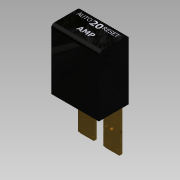
# Autodesk Inventor part: VB3-A20-F57
Saved by Autodesk Inventor 2020.1 (Build 241239000, 239)
## iProperties
Created: 2019-11-19
Part Number: VB3-A20-F57
Document SubType Name: Modeling
Designer: Autodesk Inc.
Density: 1 g/cm^3
Catalog Web Link: http://www.snapaction.net/pdf/vb3.pdf
Description: Circuit Breaker 20 Amp
Vendor: Snap Action
Material: Generic
Appearance: Glossy - Black
Category: Bag #3
Company: Autodesk Inc.
Author: Autodesk Inc.
Keywords: Black Tote
Autodesk Inventor part; units mm, degrees
note: some values were not read from the file. Chosen so that the rebuilt part matches the saved one: direction of "Emboss1"; direction of "Emboss3".
sketch "Sketch1" plane through (0, 0, 0) normal (0, 0, 1) x (1, 0, 0)
  line L0 (0, 0) -> (15.748, 0)
  line L1 (15.748, 0) -> (15.748, 9.906)
  line L2 (15.748, 9.906) -> (0, 9.906)
  line L3 (0, 9.906) -> (0, 0)
  dimension "d0" = 15.748
  dimension "d1" = 9.906
  constraints: 8 end point, 2 parallel, 1 horizontal, 1 perpendicular
  measures "d0" distance of L1.end L2.end
  measures "d1" distance of L0.end L1.end
extrude "Extrusion1" add sketch "Sketch1" against normal blind 19.812
fillet "Fillet1" radius 0.254 8 edges at (0, 0, -9.906) (15.748, 0, -9.906) (15.748, 9.906, -9.906) (0, 9.906, -9.906) (7.874, 0, -19.812) (7.874, 9.906, -19.812) (15.748, 4.953, -19.812) (0, 4.953, -19.812)
fillet "Fillet1" radius 1.27 2 edges at (7.874, 0, 0) (7.874, 9.906, 0)
sketch "Sketch2" plane through (0, 0, -19.812) normal (0, 0, -1) x (-1, 0, 0)
  line L0 (-1.0033, 8.6678) -> (-6.3881, 8.6677)
  line L1 (-6.3881, 8.6677) -> (-6.3881, 7.8803)
  line L2 (-6.3881, 7.8803) -> (-1.0033, 7.8803)
  line L3 (-1.0033, 7.8803) -> (-1.0033, 8.6678)
  line L4 (-0.254, 9.906) -> (-15.494, 9.906) projected
  line L5 (-0.254, 0.254) -> (-15.494, 0.254) projected
  line L6 (-15.494, 9.652) -> (-0.254, 9.652) projected
  line L7 (-7.874, 0.254) -> (-7.874, 9.652) construction
  point P0 (0, 0)
  dimension "d6" = 5.3848
  dimension "d8" = 0.7874
  dimension "d13" = 1.4859
  constraints: 10 end point, 2 midpoint, 2 parallel, 1 horizontal, 1 perpendicular
  measures "d6" distance of L1.end L2.end
  measures "d8" distance of L2.end L0.start
  measures "d13" distance between parallel lines of L7 L1
extrude "Extrusion3" add sketch "Sketch2" along normal blind 14.478
sketch "Sketch3" plane through (6.3881, 7.8803, -19.812) normal (1, 0, 0) x (0, 0, -1)
  line L0 (14.478, 0) -> (14.478, 0.7874) projected
  line L1 (0, 0.7874) -> (14.478, 0.7874) projected
  line L2 (0, 0) -> (14.478, 0) projected
  line L3 (13.8941, 0) -> (14.478, 0.3937)
  line L4 (13.8941, 0.7874) -> (14.478, 0.3937)
  point P0 (-19.812, -7.8803)
  constraints: 4 end point, 2 point on line, 1 midpoint
extrude "Extrusion4" cut sketch "Sketch3" against normal up to next
sketch "Sketch4" plane through (1.0033, 7.8803, -19.812) normal (0, -1, 0) x (1, 0, 0)
  line L0 (5.3848, -14.478) -> (0, -14.478) projected
  line L1 (0, -13.8941) -> (0.5839, -14.478)
  line L2 (5.3848, -13.8941) -> (4.8009, -14.478)
  line L3 (0, -13.8941) -> (0, -14.478)
  line L4 (4.8009, -14.478) -> (5.3848, -14.478)
  line L5 (5.3848, -13.8941) -> (5.3848, -14.478)
  point P0 (-1.0033, 19.812)
  dimension "d18" = 0.5839
  dimension "d19" = 0.5839
  dimension "d20" = 0.5839
  constraints: 10 end point, 3 perpendicular, 2 point on line, 1 collinear
  measures "d18" distance of L0.end L1.start
  measures "d19" distance of L1.end L0.end
  measures "d20" distance of L0.start L2.end
extrude "Extrusion5" cut sketch "Sketch4" against normal through all
ref_plane "Work Plane1" through (7.874, 1.27, 0) normal (1, 0, 0) x (0, 0, -1)
mirror "Mirror1" about plane through (7.874, 1.27, 0) normal (1, 0, 0) of "Extrusion3", "Extrusion4", "Extrusion5"
ref_plane "Work Plane2" through (0, 0, 4.7625) normal (0, 0, 1) x (1, 0, 0)
sketch "Sketch6" plane through (0, 0, 4.7625) normal (0, 0, 1) x (1, 0, 0)
  line L0 (-0.5435, 9.1913) -> (16.2915, 9.1913) construction
  line L1 (16.2915, 9.1913) -> (16.2915, 2.8312) construction
  line L2 (16.2915, 2.8312) -> (-0.5435, 2.8312) construction
  line L3 (-0.5435, 2.8312) -> (-0.5435, 9.1913) construction
  line L4 (0, 8.636) -> (15.748, 8.636) projected
  line L5 (1.2137, 7.0222) -> (1.6418, 8.2922)
  line L6 (1.6418, 8.2922) -> (1.8497, 8.2922)
  line L7 (1.8497, 8.2922) -> (2.2779, 7.0222)
  line L8 (2.2779, 7.0222) -> (2.0998, 7.0222)
  line L9 (2.0998, 7.0222) -> (1.9846, 7.3773)
  line L10 (1.9846, 7.3773) -> (1.4998, 7.3773)
  line L11 (1.4998, 7.3773) -> (1.3845, 7.0222)
  line L12 (1.3845, 7.0222) -> (1.2137, 7.0222)
  line L13 (1.9382, 7.5213) -> (1.7417, 8.1193)
  line L14 (1.7417, 8.1193) -> (1.5461, 7.5213)
  line L15 (1.5461, 7.5213) -> (1.9382, 7.5213)
  spline S0 degree 2 poles (2.8419, 6.9954) (2.7297, 6.9954) (2.563, 7.0541) (2.5043, 7.1128) knots 0 0 0 1 2 2 2
  spline S1 degree 2 poles (2.5043, 7.1128) (2.4374, 7.1786) (2.3828, 7.3639) (2.3828, 7.4997) knots 0 0 0 1 2 2 2
  line L16 (2.3828, 7.4997) -> (2.3828, 8.2922)
  line L17 (2.3828, 8.2922) -> (2.5516, 8.2922)
  line L18 (2.5516, 8.2922) -> (2.5516, 7.4997)
  spline S2 degree 2 poles (2.5516, 7.4997) (2.5516, 7.4112) (2.5743, 7.2918) (2.6062, 7.2435) knots 0 0 0 1 2 2 2
  spline S3 degree 2 poles (2.6062, 7.2435) (2.6401, 7.192) (2.7575, 7.1395) (2.8419, 7.1395) knots 0 0 0 1 2 2 2
  spline S4 degree 2 poles (2.8419, 7.1395) (2.9211, 7.1395) (3.0446, 7.192) (3.0786, 7.2435) knots 0 0 0 1 2 2 2
  spline S5 degree 2 poles (3.0786, 7.2435) (3.1105, 7.2918) (3.1331, 7.4102) (3.1331, 7.4956) knots 0 0 0 1 2 2 2
  line L19 (3.1331, 7.4956) -> (3.1331, 8.2922)
  line L20 (3.1331, 8.2922) -> (3.3019, 8.2922)
  line L21 (3.3019, 8.2922) -> (3.3019, 7.4997)
  spline S6 degree 2 poles (3.3019, 7.4997) (3.3019, 7.367) (3.2484, 7.1776) (3.1805, 7.1128) knots 0 0 0 1 2 2 2
  spline S7 degree 2 poles (3.1805, 7.1128) (3.1197, 7.0531) (2.9592, 6.9954) (2.8419, 6.9954) knots 0 0 0 1 2 2 2
  line L22 (3.8402, 7.0222) -> (3.8402, 8.1419)
  line L23 (3.8402, 8.1419) -> (3.4141, 8.1419)
  line L24 (3.4141, 8.1419) -> (3.4141, 8.2922)
  line L25 (3.4141, 8.2922) -> (4.435, 8.2922)
  line L26 (4.435, 8.2922) -> (4.435, 8.1419)
  line L27 (4.435, 8.1419) -> (4.0089, 8.1419)
  line L28 (4.0089, 8.1419) -> (4.0089, 7.0222)
  line L29 (4.0089, 7.0222) -> (3.8402, 7.0222)
  spline S8 degree 2 poles (5.4621, 8.1471) (5.5342, 8.0627) (5.6144, 7.8157) (5.6144, 7.6572) knots 0 0 0 1 2 2 2
  spline S9 degree 2 poles (5.6144, 7.6572) (5.6144, 7.5028) (5.5362, 7.2527) (5.4621, 7.1683) knots 0 0 0 1 2 2 2
  spline S10 degree 2 poles (5.4621, 7.1683) (5.3839, 7.0798) (5.1771, 6.9954) (5.0525, 6.9954) knots 0 0 0 1 2 2 2
  spline S11 degree 2 poles (5.0525, 6.9954) (4.9239, 6.9954) (4.718, 7.0829) (4.6429, 7.1683) knots 0 0 0 1 2 2 2
  spline S12 degree 2 poles (4.6429, 7.1683) (4.5698, 7.2527) (4.4916, 7.5008) (4.4916, 7.6572) knots 0 0 0 1 2 2 2
  spline S13 degree 2 poles (4.4916, 7.6572) (4.4916, 7.8167) (4.5709, 8.0596) (4.6439, 8.1471) knots 0 0 0 1 2 2 2
  spline S14 degree 2 poles (4.6439, 8.1471) (4.718, 8.2315) (4.9249, 8.319) (5.0525, 8.319) knots 0 0 0 1 2 2 2
  spline S15 degree 2 poles (5.0525, 8.319) (5.1822, 8.319) (5.3901, 8.2284) (5.4621, 8.1471) knots 0 0 0 1 2 2 2
  spline S16 degree 2 poles (5.4385, 7.6572) (5.4385, 7.7828) (5.3839, 7.9773) (5.3345, 8.0411) knots 0 0 0 1 2 2 2
  spline S17 degree 2 poles (5.3345, 8.0411) (5.2841, 8.1069) (5.1421, 8.1728) (5.0536, 8.1728) knots 0 0 0 1 2 2 2
  spline S18 degree 2 poles (5.0536, 8.1728) (4.962, 8.1728) (4.824, 8.109) (4.7716, 8.0411) knots 0 0 0 1 2 2 2
  spline S19 degree 2 poles (4.7716, 8.0411) (4.7211, 7.9762) (4.6676, 7.7807) (4.6676, 7.6572) knots 0 0 0 1 2 2 2
  spline S20 degree 2 poles (4.6676, 7.6572) (4.6676, 7.4071) (4.8776, 7.1416) (5.0536, 7.1416) knots 0 0 0 1 2 2 2
  spline S21 degree 2 poles (5.0536, 7.1416) (5.2295, 7.1416) (5.4385, 7.4071) (5.4385, 7.6572) knots 0 0 0 1 2 2 2
  line L30 (10.6008, 7.0222) -> (10.3816, 7.0222)
  line L31 (10.3816, 7.0222) -> (9.9802, 7.5275)
  line L32 (9.9802, 7.5275) -> (9.7867, 7.5275)
  line L33 (9.7867, 7.5275) -> (9.7867, 7.0222)
  line L34 (9.7867, 7.0222) -> (9.6179, 7.0222)
  line L35 (9.6179, 7.0222) -> (9.6179, 8.2922)
  line L36 (9.6179, 8.2922) -> (9.9452, 8.2922)
  spline S22 degree 2 poles (9.9452, 8.2922) (10.0543, 8.2922) (10.2015, 8.2685) (10.2684, 8.2253) knots 0 0 0 1 2 2 2
  spline S23 degree 2 poles (10.2684, 8.2253) (10.3353, 8.1821) (10.4125, 8.0473) (10.4125, 7.9474) knots 0 0 0 1 2 2 2
  spline S24 degree 2 poles (10.4125, 7.9474) (10.4125, 7.8085) (10.2704, 7.6201) (10.149, 7.5749) knots 0 0 0 1 2 2 2
  line L37 (10.149, 7.5749) -> (10.6008, 7.0222)
  spline S25 degree 2 poles (10.2365, 7.934) (10.2365, 7.9896) (10.1974, 8.075) (10.1562, 8.1028) knots 0 0 0 1 2 2 2
  spline S26 degree 2 poles (10.1562, 8.1028) (10.1202, 8.1265) (10.0245, 8.1461) (9.9545, 8.1461) knots 0 0 0 1 2 2 2
  line L38 (9.9545, 8.1461) -> (9.7867, 8.1461)
  line L39 (9.7867, 8.1461) -> (9.7867, 7.6685)
  line L40 (9.7867, 7.6685) -> (9.9349, 7.6685)
  spline S27 degree 2 poles (9.9349, 7.6685) (10.008, 7.6685) (10.1243, 7.6942) (10.1644, 7.7344) knots 0 0 0 1 2 2 2
  spline S28 degree 2 poles (10.1644, 7.7344) (10.2015, 7.7694) (10.2365, 7.8682) (10.2365, 7.934) knots 0 0 0 1 2 2 2
  line L41 (10.7017, 7.0222) -> (10.7017, 8.2922)
  line L42 (10.7017, 8.2922) -> (11.4962, 8.2922)
  line L43 (11.4962, 8.2922) -> (11.4962, 8.1419)
  line L44 (11.4962, 8.1419) -> (10.8704, 8.1419)
  line L45 (10.8704, 8.1419) -> (10.8704, 7.7941)
  line L46 (10.8704, 7.7941) -> (11.454, 7.7941)
  line L47 (11.454, 7.7941) -> (11.454, 7.6438)
  line L48 (11.454, 7.6438) -> (10.8704, 7.6438)
  line L49 (10.8704, 7.6438) -> (10.8704, 7.1725)
  line L50 (10.8704, 7.1725) -> (11.4962, 7.1725)
  line L51 (11.4962, 7.1725) -> (11.4962, 7.0222)
  line L52 (11.4962, 7.0222) -> (10.7017, 7.0222)
  spline S29 degree 2 poles (12.0355, 6.9996) (11.8976, 6.9996) (11.7041, 7.0572) (11.6186, 7.0984) knots 0 0 0 1 2 2 2
  line L53 (11.6186, 7.0984) -> (11.6186, 7.3104)
  line L54 (11.6186, 7.3104) -> (11.631, 7.3104)
  spline S30 degree 2 poles (11.631, 7.3104) (11.7144, 7.2321) (11.9253, 7.1457) (12.0231, 7.1457) knots 0 0 0 1 2 2 2
  spline S31 degree 2 poles (12.0231, 7.1457) (12.1631, 7.1457) (12.3061, 7.262) (12.3061, 7.3577) knots 0 0 0 1 2 2 2
  spline S32 degree 2 poles (12.3061, 7.3577) (12.3061, 7.4339) (12.231, 7.5285) (12.1497, 7.5522) knots 0 0 0 1 2 2 2
  spline S33 degree 2 poles (12.1497, 7.5522) (12.091, 7.5687) (11.9933, 7.5913) (11.9202, 7.6099) knots 0 0 0 1 2 2 2
  spline S34 degree 2 poles (11.9202, 7.6099) (11.8543, 7.6273) (11.7504, 7.6798) (11.7102, 7.722) knots 0 0 0 1 2 2 2
  spline S35 degree 2 poles (11.7102, 7.722) (11.6711, 7.7642) (11.6279, 7.8774) (11.6279, 7.9515) knots 0 0 0 1 2 2 2
  spline S36 degree 2 poles (11.6279, 7.9515) (11.6279, 8.1059) (11.8687, 8.3148) (12.055, 8.3148) knots 0 0 0 1 2 2 2
  spline S37 degree 2 poles (12.055, 8.3148) (12.1621, 8.3148) (12.3514, 8.2726) (12.4327, 8.2325) knots 0 0 0 1 2 2 2
  line L55 (12.4327, 8.2325) -> (12.4327, 8.0308)
  line L56 (12.4327, 8.0308) -> (12.4204, 8.0308)
  spline S38 degree 2 poles (12.4204, 8.0308) (12.3597, 8.0864) (12.1703, 8.1687) (12.0663, 8.1687) knots 0 0 0 1 2 2 2
  spline S39 degree 2 poles (12.0663, 8.1687) (11.949, 8.1687) (11.8039, 8.0586) (11.8039, 7.969) knots 0 0 0 1 2 2 2
  spline S40 degree 2 poles (11.8039, 7.969) (11.8039, 7.8888) (11.8893, 7.793) (11.9696, 7.7714) knots 0 0 0 1 2 2 2
  spline S41 degree 2 poles (11.9696, 7.7714) (12.0231, 7.757) (12.1785, 7.72) (12.23, 7.7045) knots 0 0 0 1 2 2 2
  spline S42 degree 2 poles (12.23, 7.7045) (12.3607, 7.6644) (12.4821, 7.5028) (12.4821, 7.3845) knots 0 0 0 1 2 2 2
  spline S43 degree 2 poles (12.4821, 7.3845) (12.4821, 7.3093) (12.4214, 7.1653) (12.3669, 7.1148) knots 0 0 0 1 2 2 2
  spline S44 degree 2 poles (12.3669, 7.1148) (12.3061, 7.0592) (12.1518, 6.9996) (12.0355, 6.9996) knots 0 0 0 1 2 2 2
  line L57 (12.654, 7.0222) -> (12.654, 8.2922)
  line L58 (12.654, 8.2922) -> (13.4485, 8.2922)
  line L59 (13.4485, 8.2922) -> (13.4485, 8.1419)
  line L60 (13.4485, 8.1419) -> (12.8228, 8.1419)
  line L61 (12.8228, 8.1419) -> (12.8228, 7.7941)
  line L62 (12.8228, 7.7941) -> (13.4063, 7.7941)
  line L63 (13.4063, 7.7941) -> (13.4063, 7.6438)
  line L64 (13.4063, 7.6438) -> (12.8228, 7.6438)
  line L65 (12.8228, 7.6438) -> (12.8228, 7.1725)
  line L66 (12.8228, 7.1725) -> (13.4485, 7.1725)
  line L67 (13.4485, 7.1725) -> (13.4485, 7.0222)
  line L68 (13.4485, 7.0222) -> (12.654, 7.0222)
  line L69 (13.9302, 7.0222) -> (13.9302, 8.1419)
  line L70 (13.9302, 8.1419) -> (13.5041, 8.1419)
  line L71 (13.5041, 8.1419) -> (13.5041, 8.2922)
  line L72 (13.5041, 8.2922) -> (14.525, 8.2922)
  line L73 (14.525, 8.2922) -> (14.525, 8.1419)
  line L74 (14.525, 8.1419) -> (14.099, 8.1419)
  line L75 (14.099, 8.1419) -> (14.099, 7.0222)
  line L76 (14.099, 7.0222) -> (13.9302, 7.0222)
  line L77 (5.3299, 2.8312) -> (5.8878, 4.4822)
  line L78 (5.8878, 4.4822) -> (6.3401, 4.4822)
  line L79 (6.3401, 4.4822) -> (6.898, 2.8312)
  line L80 (6.898, 2.8312) -> (6.4712, 2.8312)
  line L81 (6.4712, 2.8312) -> (6.3682, 3.1684)
  line L82 (6.3682, 3.1684) -> (5.8491, 3.1684)
  line L83 (5.8491, 3.1684) -> (5.7447, 2.8312)
  line L84 (5.7447, 2.8312) -> (5.3299, 2.8312)
  line L85 (6.2772, 3.468) -> (6.1086, 4.0139)
  line L86 (6.1086, 4.0139) -> (5.9387, 3.468)
  line L87 (5.9387, 3.468) -> (6.2772, 3.468)
  line L88 (8.7483, 2.8312) -> (8.3363, 2.8312)
  line L89 (8.3363, 2.8312) -> (8.3363, 3.9256)
  line L90 (8.3363, 3.9256) -> (8.0366, 3.2192)
  line L91 (8.0366, 3.2192) -> (7.7529, 3.2192)
  line L92 (7.7529, 3.2192) -> (7.4532, 3.9256)
  line L93 (7.4532, 3.9256) -> (7.4532, 2.8312)
  line L94 (7.4532, 2.8312) -> (7.0625, 2.8312)
  line L95 (7.0625, 2.8312) -> (7.0625, 4.4822)
  line L96 (7.0625, 4.4822) -> (7.5402, 4.4822)
  line L97 (7.5402, 4.4822) -> (7.9068, 3.6674)
  line L98 (7.9068, 3.6674) -> (8.2707, 4.4822)
  line L99 (8.2707, 4.4822) -> (8.7483, 4.4822)
  line L100 (8.7483, 4.4822) -> (8.7483, 2.8312)
  spline S45 degree 2 poles (10.3605, 3.9617) (10.3605, 3.8467) (10.2869, 3.638) (10.2187, 3.5684) knots 0 0 0 1 2 2 2
  spline S46 degree 2 poles (10.2187, 3.5684) (10.1772, 3.5242) (10.0756, 3.452) (10.0153, 3.4266) knots 0 0 0 1 2 2 2
  spline S47 degree 2 poles (10.0153, 3.4266) (9.9538, 3.4012) (9.8106, 3.3717) (9.7223, 3.3717) knots 0 0 0 1 2 2 2
  line L101 (9.7223, 3.3717) -> (9.5056, 3.3717)
  line L102 (9.5056, 3.3717) -> (9.5056, 2.8312)
  line L103 (9.5056, 2.8312) -> (9.0908, 2.8312)
  line L104 (9.0908, 2.8312) -> (9.0908, 4.4822)
  line L105 (9.0908, 4.4822) -> (9.7317, 4.4822)
  spline S48 degree 2 poles (9.7317, 4.4822) (9.8735, 4.4822) (10.0809, 4.43) (10.1652, 4.3738) knots 0 0 0 1 2 2 2
  spline S49 degree 2 poles (10.1652, 4.3738) (10.2589, 4.3109) (10.3605, 4.1049) (10.3605, 3.9617) knots 0 0 0 1 2 2 2
  spline S50 degree 2 poles (9.9351, 3.951) (9.9351, 4.0219) (9.8682, 4.1223) (9.8227, 4.141) knots 0 0 0 1 2 2 2
  spline S51 degree 2 poles (9.8227, 4.141) (9.7638, 4.1664) (9.6568, 4.1745) (9.5645, 4.1745) knots 0 0 0 1 2 2 2
  line L106 (9.5645, 4.1745) -> (9.5056, 4.1745)
  line L107 (9.5056, 4.1745) -> (9.5056, 3.6794)
  line L108 (9.5056, 3.6794) -> (9.535, 3.6794)
  spline S52 degree 2 poles (9.535, 3.6794) (9.5926, 3.6794) (9.6969, 3.6821) (9.7357, 3.6888) knots 0 0 0 1 2 2 2
  spline S53 degree 2 poles (9.7357, 3.6888) (9.7692, 3.6942) (9.8428, 3.7263) (9.8628, 3.7463) knots 0 0 0 1 2 2 2
  spline S54 degree 2 poles (9.8628, 3.7463) (9.9056, 3.7865) (9.9351, 3.8761) (9.9351, 3.951) knots 0 0 0 1 2 2 2
  point P0 (0, 0)
  point P1 (7.874, 9.1913)
  point P2 (7.874, 8.636)
  constraints: 2 midpoint, 1 vertical alignment, 2 other
emboss "Emboss1" sketch "Sketch6" operation cut depth 0.0025 direction (0, 0, -1)
ref_plane "Work Plane4" through (0, 0, 4.7625) normal (0, 0, 1) x (1, 0, 0)
sketch "Sketch8" plane through (0, 0, 4.7625) normal (0, 0, 1) x (1, 0, 0)
  line L0 (5.8091, 8.4478) -> (9.9389, 8.4478) construction
  line L1 (9.9389, 8.4478) -> (9.9389, 2.3778) construction
  line L2 (9.9389, 2.3778) -> (5.8091, 2.3778) construction
  line L3 (5.8091, 2.3778) -> (5.8091, 8.4478) construction
  line L4 (0, 8.636) -> (15.748, 8.636) projected
  line L5 (7.5084, 6.3747) -> (6.0149, 6.3747)
  line L6 (6.0149, 6.3747) -> (6.0149, 6.7056)
  spline S0 degree 2 poles (6.0149, 6.7056) (6.2043, 6.8571) (6.5072, 7.1239) (6.6209, 7.2441) knots 0 0 0 1 2 2 2
  spline S1 degree 2 poles (6.6209, 7.2441) (6.7707, 7.4005) (6.9041, 7.6393) (6.9041, 7.7645) knots 0 0 0 1 2 2 2
  spline S2 degree 2 poles (6.9041, 7.7645) (6.9041, 7.9061) (6.7345, 8.0576) (6.583, 8.0576) knots 0 0 0 1 2 2 2
  spline S3 degree 2 poles (6.583, 8.0576) (6.5056, 8.0576) (6.3673, 8.0197) (6.2965, 7.99) knots 0 0 0 1 2 2 2
  spline S4 degree 2 poles (6.2965, 7.99) (6.2273, 7.9588) (6.1285, 7.8929) (6.1038, 7.8764) knots 0 0 0 1 2 2 2
  line L7 (6.1038, 7.8764) -> (6.0643, 7.8764)
  line L8 (6.0643, 7.8764) -> (6.0643, 8.3194)
  spline S5 degree 2 poles (6.0643, 8.3194) (6.1499, 8.3605) (6.5155, 8.4462) (6.6851, 8.4462) knots 0 0 0 1 2 2 2
  spline S6 degree 2 poles (6.6851, 8.4462) (7.0474, 8.4462) (7.4195, 8.1234) (7.4195, 7.832) knots 0 0 0 1 2 2 2
  spline S7 degree 2 poles (7.4195, 7.832) (7.4195, 7.6525) (7.2499, 7.3067) (7.0539, 7.1091) knots 0 0 0 1 2 2 2
  spline S8 degree 2 poles (7.0539, 7.1091) (6.9304, 6.9872) (6.6983, 6.7979) (6.6472, 6.7583) knots 0 0 0 1 2 2 2
  line L9 (6.6472, 6.7583) -> (7.5084, 6.7583)
  line L10 (7.5084, 6.7583) -> (7.5084, 6.3747)
  spline S9 degree 2 poles (9.2621, 7.3907) (9.2621, 7.1272) (9.1782, 6.732) (9.0843, 6.5986) knots 0 0 0 1 2 2 2
  spline S10 degree 2 poles (9.0843, 6.5986) (8.9921, 6.4669) (8.694, 6.3318) (8.48, 6.3318) knots 0 0 0 1 2 2 2
  spline S11 degree 2 poles (8.48, 6.3318) (8.2643, 6.3318) (7.9679, 6.4669) (7.874, 6.6019) knots 0 0 0 1 2 2 2
  spline S12 degree 2 poles (7.874, 6.6019) (7.7801, 6.7353) (7.6961, 7.1272) (7.6961, 7.3907) knots 0 0 0 1 2 2 2
  spline S13 degree 2 poles (7.6961, 7.3907) (7.6961, 7.6607) (7.7801, 8.0427) (7.8756, 8.1811) knots 0 0 0 1 2 2 2
  spline S14 degree 2 poles (7.8756, 8.1811) (7.9711, 8.3161) (8.2725, 8.4478) (8.48, 8.4478) knots 0 0 0 1 2 2 2
  spline S15 degree 2 poles (8.48, 8.4478) (8.699, 8.4478) (8.9921, 8.3095) (9.0859, 8.1728) knots 0 0 0 1 2 2 2
  spline S16 degree 2 poles (9.0859, 8.1728) (9.1782, 8.0394) (9.2621, 7.6459) (9.2621, 7.3907) knots 0 0 0 1 2 2 2
  spline S17 degree 2 poles (8.75, 7.3907) (8.75, 7.7677) (8.6265, 8.0724) (8.48, 8.0724) knots 0 0 0 1 2 2 2
  spline S18 degree 2 poles (8.48, 8.0724) (8.3334, 8.0724) (8.2083, 7.7677) (8.2083, 7.389) knots 0 0 0 1 2 2 2
  spline S19 degree 2 poles (8.2083, 7.389) (8.2083, 7.0169) (8.3334, 6.7073) (8.48, 6.7073) knots 0 0 0 1 2 2 2
  spline S20 degree 2 poles (8.48, 6.7073) (8.6249, 6.7073) (8.75, 7.0169) (8.75, 7.3907) knots 0 0 0 1 2 2 2
  point P0 (0, 0)
  point P1 (7.874, 8.4478)
  point P2 (7.874, 8.636)
  constraints: 2 midpoint, 1 vertical alignment, 2 other
emboss "Emboss3" sketch "Sketch8" operation cut depth 0.0025 direction (0, 0, -1)
equation "\"d19\" = d18"
body "Solid1"
